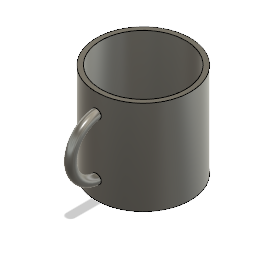
水杯 (Autodesk Fusion 360 design; units mm, degrees)
Autodesk Fusion 360 part; units mm, degrees
sphere "球体基本要素1" add diameter 8 placed x (1, 0, 0) y (0, 0, -1) z (0, 1, 0) at (15, 0, -25) makes body 1
move_body "对齐1" bodies 1 to x (1, 0, 0) y (0, 1, 0) z (0, 0, 1) at (-15, 30, 55)
combine "合并1" [no effect]
delete_face "删除面1" 1 faces at (3.7923, 30.9455, 29.1489) on bodies 1
cylinder "圆柱体基本要素3" add diameter 20 height 20 placed x (1, 0, 0) y (0, 0, -1) z (0, 1, 0) at (0, 0, 0) separate body makes body 2
cylinder "圆柱体基本要素4" add diameter 18 height 20 placed x (1, 0, 0) y (0, 0, -1) z (0, 1, 0) at (50, 0, 0) separate body makes body 3
torus "圆环体基本要素1" add centre line diameter 12 section diameter 2 placed x (0, 0, -1) y (0, 1, 0) z (1, 0, 0) at (0, 40, 60) separate body makes body 4
move_body "MoveFace1" bodies 4 to x (1, 0, 0) y (0, 1, 0) z (0, 0, 1) at (-16, 0, -23) on bodies 4
move_body "移动1" bodies 4 to x (1, 0, 0) y (0, 1, 0) z (0, 0, 1) at (16, 0, 0)
move_body "MoveFace2" bodies 4 to x (1, 0, 0) y (0, 1, 0) z (0, 0, 1) at (0, -30, -27.5) on bodies 4
combine "合并2" operation add target body 2 tool bodies 4
move_body "对齐3" bodies 3 to x (1, 0, 0) y (0, 1, 0) z (0, 0, 1) at (-50, 0, 0)
move_face "偏移面1" offset -2 1 faces at (-5.1676, 0, -0.3267) on bodies 3
combine "合并3" operation cut target body 2 tool bodies 3
